Autodesk Inventor part; units mm, degrees
(part 2 of 2)
  line L486 (-92.9242, 137.6382) -> (-92.9242, 136.9026) construction
  line L487 (-92.9242, 136.9026) -> (-86.3376, 126.2158) construction
  line L488 (-86.3376, 126.2158) -> (-85.8147, 126.2158) construction
  line L489 (-85.8147, 126.2158) -> (-86.0963, 127.2615) construction
  line L490 (-86.0963, 127.2615) -> (-92.2499, 139.3275) construction
  line L491 (-92.2499, 139.3275) -> (-96.1914, 145.3604) construction
  line L492 (-96.1914, 145.3604) -> (-96.6339, 145.642) construction
  line L493 (-96.6339, 145.642) -> (-99.1677, 146.7681) construction
  line L494 (-99.1677, 146.7681) -> (-105.7825, 149.6506) construction
  spline S7 degree 4 poles (-105.7825, 149.6506) (-98.5638, 144.2366) (-96.1387, 141.0784) (-92.9242, 137.6382) (-92.9242, 136.9026) (-86.3376, 126.2158) (-85.8147, 126.2158) (-86.0963, 127.2615) (-92.2499, 139.3275) (-96.1914, 145.3604) (-96.6339, 145.642) (-99.1677, 146.7681) (-105.7825, 149.6506) knots 1 1 1 1 1 2 3 4 5 6 7 8 9 10 10 10 10 10
  line L495 (-151.4576, 116.9137) -> (-151.4576, 113.6219)
  line L496 (-232.8904, 100.9083) -> (-224.086, 105.444) construction
  line L497 (-224.086, 105.444) -> (-217.8517, 107.8081) construction
  line L498 (-217.8517, 107.8081) -> (-210.9325, 109.9735) construction
  line L499 (-210.9325, 109.9735) -> (-204.045, 111.8416) construction
  line L500 (-204.045, 111.8416) -> (-196.96, 113.1781) construction
  line L501 (-196.96, 113.1781) -> (-181.3524, 115.2983) construction
  line L502 (-181.3524, 115.2983) -> (-172.7322, 116.2018) construction
  line L503 (-172.7322, 116.2018) -> (-164.4787, 116.6804) construction
  line L504 (-164.4787, 116.6804) -> (-155.3689, 116.9137) construction
  line L505 (-155.3689, 116.9137) -> (-151.4576, 116.9137) construction
  spline S8 degree 4 poles (-232.8904, 100.9083) (-224.086, 105.444) (-217.8517, 107.8081) (-210.9325, 109.9735) (-204.045, 111.8416) (-196.96, 113.1781) (-181.3524, 115.2983) (-172.7322, 116.2018) (-164.4787, 116.6804) (-155.3689, 116.9137) (-151.4576, 116.9137) knots 1 1 1 1 1 2 3 4 5 6 7 8 8 8 8 8
  line L506 (-151.4576, 113.6219) -> (-160.6161, 113.6219) construction
  line L507 (-160.6161, 113.6219) -> (-167.753, 113.3145) construction
  line L508 (-167.753, 113.3145) -> (-176.028, 112.8336) construction
  line L509 (-176.028, 112.8336) -> (-190.3891, 111.4372) construction
  line L510 (-190.3891, 111.4372) -> (-200.0112, 109.6691) construction
  line L511 (-200.0112, 109.6691) -> (-210.3251, 107.9445) construction
  line L512 (-210.3251, 107.9445) -> (-217.922, 106.0369) construction
  line L513 (-217.922, 106.0369) -> (-223.8067, 104.1386) construction
  line L514 (-223.8067, 104.1386) -> (-227.183, 102.909) construction
  line L515 (-227.183, 102.909) -> (-229.6689, 101.9664) construction
  line L516 (-229.6689, 101.9664) -> (-232.2744, 101.1419) construction
  line L517 (-232.2744, 101.1419) -> (-232.8904, 100.9083) construction
  spline S9 degree 4 poles (-151.4576, 113.6219) (-160.6161, 113.6219) (-167.753, 113.3145) (-176.028, 112.8336) (-190.3891, 111.4372) (-200.0112, 109.6691) (-210.3251, 107.9445) (-217.922, 106.0369) (-223.8067, 104.1386) (-227.183, 102.909) (-229.6689, 101.9664) (-232.2744, 101.1419) (-232.8904, 100.9083) knots 1 1 1 1 1 2 3 4 5 6 7 8 9 10 10 10 10 10
  line L518 (-201.4615, 98.1456) -> (-198.4129, 100.8521) construction
  line L519 (-198.4129, 100.8521) -> (-196.3192, 102.3711) construction
  line L520 (-196.3192, 102.3711) -> (-194.2664, 103.5238) construction
  line L521 (-194.2664, 103.5238) -> (-191.3421, 104.8481) construction
  line L522 (-191.3421, 104.8481) -> (-187.3069, 106.5757) construction
  line L523 (-187.3069, 106.5757) -> (-184.015, 107.9604) construction
  line L524 (-184.015, 107.9604) -> (-181.0006, 109.0583) construction
  line L525 (-181.0006, 109.0583) -> (-179.1462, 109.7366) construction
  line L526 (-179.1462, 109.7366) -> (-174.5466, 111.2151) construction
  line L527 (-174.5466, 111.2151) -> (-172.2748, 111.8831) construction
  line L528 (-172.2748, 111.8831) -> (-171.1664, 112.1657) construction
  spline S10 degree 4 poles (-201.4615, 98.1456) (-198.4129, 100.8521) (-196.3192, 102.3711) (-194.2664, 103.5238) (-191.3421, 104.8481) (-187.3069, 106.5757) (-184.015, 107.9604) (-181.0006, 109.0583) (-179.1462, 109.7366) (-174.5466, 111.2151) (-172.2748, 111.8831) (-171.1664, 112.1657) knots 1 1 1 1 1 2 3 4 5 6 7 8 9 9 9 9 9
  line L529 (-171.1664, 112.1657) -> (-174.7868, 110.3396) construction
  line L530 (-174.7868, 110.3396) -> (-176.4505, 109.5236) construction
  line L531 (-176.4505, 109.5236) -> (-178.3607, 108.6636) construction
  line L532 (-178.3607, 108.6636) -> (-180.8153, 107.389) construction
  line L533 (-180.8153, 107.389) -> (-182.668, 106.5757) construction
  line L534 (-182.668, 106.5757) -> (-184.7906, 105.4752) construction
  line L535 (-184.7906, 105.4752) -> (-188.8328, 103.7438) construction
  line L536 (-188.8328, 103.7438) -> (-192.9088, 101.6116) construction
  line L537 (-192.9088, 101.6116) -> (-201.4615, 98.1456) construction
  spline S11 degree 4 poles (-171.1664, 112.1657) (-174.7868, 110.3396) (-176.4505, 109.5236) (-178.3607, 108.6636) (-180.8153, 107.389) (-182.668, 106.5757) (-184.7906, 105.4752) (-188.8328, 103.7438) (-192.9088, 101.6116) (-201.4615, 98.1456) knots 1 1 1 1 1 2 3 4 5 6 7 7 7 7 7
  line L538 (-175.3989, 90.8936) -> (-175.0678, 91.6636) construction
  line L539 (-167.9379, 100.2753) -> (-166.4649, 101.6772) construction
  line L540 (-166.4649, 101.6772) -> (-163.3138, 104.358) construction
  line L541 (-163.3138, 104.358) -> (-160.8042, 106.4947) construction
  line L542 (-160.8042, 106.4947) -> (-158.3215, 108.2959) construction
  line L543 (-158.3215, 108.2959) -> (-156.8552, 109.3592) construction
  line L544 (-156.8552, 109.3592) -> (-154.7761, 110.5531) construction
  spline S12 degree 4 poles (-175.3989, 90.8936) (-175.0678, 91.6636) (-174.5782, 92.4731) (-173.7131, 93.7871) (-171.7339, 96.3811) (-169.8583, 98.3242) (-167.9379, 100.2753) (-166.4649, 101.6772) (-163.3138, 104.358) (-160.8042, 106.4947) (-158.3215, 108.2959) (-156.8552, 109.3592) (-154.7761, 110.5531) knots 1 1 1 1 1 1.158039 1.166811 1.450335 2 3 4 5 6 7 7 7 7 7
  line L545 (-175.3989, 90.8936) -> (-172.1206, 94.0179) construction
  line L546 (-172.1206, 94.0179) -> (-168.4171, 97.5439) construction
  line L547 (-168.4171, 97.5439) -> (-165.0932, 101.0251) construction
  line L548 (-165.0932, 101.0251) -> (-161.4603, 104.2831) construction
  line L549 (-161.4603, 104.2831) -> (-159.6446, 105.8928) construction
  line L550 (-159.6446, 105.8928) -> (-157.3682, 108.0729) construction
  line L551 (-157.3682, 108.0729) -> (-154.7761, 110.5531) construction
  spline S13 degree 4 poles (-175.3989, 90.8936) (-172.1206, 94.0179) (-168.4171, 97.5439) (-165.0932, 101.0251) (-161.4603, 104.2831) (-159.6446, 105.8928) (-157.3682, 108.0729) (-154.7761, 110.5531) knots 1 1 1 1 1 2 3 4 5 5 5 5 5
  line L552 (-175.0678, 91.6636) -> (-174.5782, 92.4731) construction
  line L553 (-169.8583, 98.3242) -> (-167.9379, 100.2753) construction
  line L554 (-174.5782, 92.4731) -> (-173.7131, 93.7871) construction
  line L555 (-173.7131, 93.7871) -> (-171.7339, 96.3811) construction
  line L556 (-171.7339, 96.3811) -> (-169.8583, 98.3242) construction
  line L557 (-151.4576, 103.7438) -> (-159.2171, 103.7438) construction
  line L558 (-159.2171, 103.7438) -> (-161.5118, 103.8212) construction
  line L559 (-161.5118, 103.8212) -> (-165.7493, 103.995) construction
  line L560 (-165.7493, 103.995) -> (-174.3234, 104.7988) construction
  line L561 (-174.3234, 104.7988) -> (-183.963, 105.7115) construction
  line L562 (-183.963, 105.7115) -> (-192.1813, 106.8081) construction
  line L563 (-192.1813, 106.8081) -> (-200.9668, 108.2959) construction
  line L564 (-200.9668, 108.2959) -> (-205.9243, 109.313) construction
  spline S14 degree 4 poles (-151.4576, 103.7438) (-159.2171, 103.7438) (-161.5118, 103.8212) (-165.7493, 103.995) (-174.3234, 104.7988) (-183.963, 105.7115) (-192.1813, 106.8081) (-200.9668, 108.2959) (-205.9243, 109.313) knots 1 1 1 1 1 2 3 4 5 6 6 6 6 6
  line L565 (-205.9243, 109.313) -> (-206.0734, 108.8908) construction
  line L566 (-206.0734, 108.8908) -> (-205.7492, 108.8908) construction
  line L567 (-205.7492, 108.8908) -> (-204.6748, 108.4348) construction
  line L568 (-204.6748, 108.4348) -> (-201.8623, 107.6091) construction
  line L569 (-201.8623, 107.6091) -> (-199.298, 106.9147) construction
  line L570 (-199.298, 106.9147) -> (-194.7707, 106.0254) construction
  line L571 (-194.7707, 106.0254) -> (-191.951, 105.5403) construction
  line L572 (-191.951, 105.5403) -> (-189.8785, 105.1889) construction
  line L573 (-189.8785, 105.1889) -> (-183.7764, 104.1859) construction
  line L574 (-183.7764, 104.1859) -> (-176.1265, 103.3428) construction
  line L575 (-176.1265, 103.3428) -> (-169.656, 102.8387) construction
  line L576 (-169.656, 102.8387) -> (-165.7493, 102.5809) construction
  line L577 (-165.7493, 102.5809) -> (-160.6663, 102.3711) construction
  line L578 (-160.6663, 102.3711) -> (-154.8757, 102.2382) construction
  line L579 (-154.8757, 102.2382) -> (-151.4576, 102.2382) construction
  spline S15 degree 4 poles (-205.9243, 109.313) (-206.0734, 108.8908) (-205.7492, 108.8908) (-204.6748, 108.4348) (-201.8623, 107.6091) (-199.298, 106.9147) (-194.7707, 106.0254) (-191.951, 105.5403) (-189.8785, 105.1889) (-183.7764, 104.1859) (-176.1265, 103.3428) (-169.656, 102.8387) (-165.7493, 102.5809) (-160.6663, 102.3711) (-154.8757, 102.2382) (-151.4576, 102.2382) knots 1 1 1 1 1 2 3 4 5 6 7 8 9 10 11 12 13 13 13 13 13
  line L580 (-151.4576, 103.7438) -> (-151.4576, 102.2382)
  line L581 (-118.9522, 105.7115) -> (-110.734, 106.8081) construction
  spline S16 degree 4 poles (-151.4576, 103.7438) (-143.6982, 103.7438) (-141.4035, 103.8212) (-137.166, 103.995) (-128.5918, 104.7988) (-118.9522, 105.7115) (-110.734, 106.8081) (-101.9485, 108.2959) (-96.991, 109.313) knots 1 1 1 1 1 2 3 4 5 6 6 6 6 6
  line L582 (-151.4576, 103.7438) -> (-143.6982, 103.7438) construction
  line L583 (-143.6982, 103.7438) -> (-141.4035, 103.8212) construction
  line L584 (-141.4035, 103.8212) -> (-137.166, 103.995) construction
  line L585 (-137.166, 103.995) -> (-128.5918, 104.7988) construction
  line L586 (-128.5918, 104.7988) -> (-118.9522, 105.7115) construction
  line L587 (-110.734, 106.8081) -> (-101.9485, 108.2959) construction
  line L588 (-101.9485, 108.2959) -> (-96.991, 109.313) construction
  line L589 (-110.9642, 105.5403) -> (-113.0367, 105.1889) construction
  spline S17 degree 4 poles (-96.991, 109.313) (-96.8419, 108.8908) (-97.1661, 108.8908) (-98.2405, 108.4348) (-101.053, 107.6091) (-103.6172, 106.9147) (-108.1446, 106.0254) (-110.9642, 105.5403) (-113.0367, 105.1889) (-119.1389, 104.1859) (-126.7887, 103.3428) (-133.2593, 102.8387) (-137.166, 102.5809) (-142.249, 102.3711) (-148.0396, 102.2382) (-151.4576, 102.2382) knots 1 1 1 1 1 2 3 4 5 6 7 8 9 10 11 12 13 13 13 13 13
  line L590 (-96.991, 109.313) -> (-96.8419, 108.8908) construction
  line L591 (-96.8419, 108.8908) -> (-97.1661, 108.8908) construction
  line L592 (-97.1661, 108.8908) -> (-98.2405, 108.4348) construction
  line L593 (-98.2405, 108.4348) -> (-101.053, 107.6091) construction
  line L594 (-101.053, 107.6091) -> (-103.6172, 106.9147) construction
  line L595 (-103.6172, 106.9147) -> (-108.1446, 106.0254) construction
  line L596 (-108.1446, 106.0254) -> (-110.9642, 105.5403) construction
  line L597 (-113.0367, 105.1889) -> (-119.1389, 104.1859) construction
  line L598 (-119.1389, 104.1859) -> (-126.7887, 103.3428) construction
  line L599 (-126.7887, 103.3428) -> (-133.2593, 102.8387) construction
  line L600 (-133.2593, 102.8387) -> (-137.166, 102.5809) construction
  line L601 (-137.166, 102.5809) -> (-142.249, 102.3711) construction
  line L602 (-142.249, 102.3711) -> (-148.0396, 102.2382) construction
  line L603 (-148.0396, 102.2382) -> (-151.4576, 102.2382) construction
  spline S18 degree 4 poles (-151.4576, 113.6219) (-142.2991, 113.6219) (-135.1622, 113.3145) (-126.8873, 112.8336) (-112.5261, 111.4372) (-102.904, 109.6691) (-92.5902, 107.9445) (-84.9933, 106.0369) (-79.1085, 104.1386) (-75.7322, 102.909) (-73.2463, 101.9664) (-70.6409, 101.1419) (-70.0249, 100.9083) knots 1 1 1 1 1 2 3 4 5 6 7 8 9 10 10 10 10 10
  line L604 (-151.4576, 113.6219) -> (-142.2991, 113.6219) construction
  line L605 (-142.2991, 113.6219) -> (-135.1622, 113.3145) construction
  line L606 (-135.1622, 113.3145) -> (-126.8873, 112.8336) construction
  line L607 (-126.8873, 112.8336) -> (-112.5261, 111.4372) construction
  line L608 (-112.5261, 111.4372) -> (-102.904, 109.6691) construction
  line L609 (-102.904, 109.6691) -> (-92.5902, 107.9445) construction
  line L610 (-92.5902, 107.9445) -> (-84.9933, 106.0369) construction
  line L611 (-84.9933, 106.0369) -> (-79.1085, 104.1386) construction
  line L612 (-79.1085, 104.1386) -> (-75.7322, 102.909) construction
  line L613 (-75.7322, 102.909) -> (-73.2463, 101.9664) construction
  line L614 (-73.2463, 101.9664) -> (-70.6409, 101.1419) construction
  line L615 (-70.6409, 101.1419) -> (-70.0249, 100.9083) construction
  line L616 (-105.9552, 113.1781) -> (-121.5628, 115.2983) construction
  spline S19 degree 4 poles (-70.0249, 100.9083) (-78.8293, 105.444) (-85.0636, 107.8081) (-91.9828, 109.9735) (-98.8702, 111.8416) (-105.9552, 113.1781) (-121.5628, 115.2983) (-130.183, 116.2018) (-138.4365, 116.6804) (-147.5463, 116.9137) (-151.4576, 116.9137) knots 1 1 1 1 1 2 3 4 5 6 7 8 8 8 8 8
  line L617 (-70.0249, 100.9083) -> (-78.8293, 105.444) construction
  line L618 (-78.8293, 105.444) -> (-85.0636, 107.8081) construction
  line L619 (-85.0636, 107.8081) -> (-91.9828, 109.9735) construction
  line L620 (-91.9828, 109.9735) -> (-98.8702, 111.8416) construction
  line L621 (-98.8702, 111.8416) -> (-105.9552, 113.1781) construction
  line L622 (-121.5628, 115.2983) -> (-130.183, 116.2018) construction
  line L623 (-130.183, 116.2018) -> (-138.4365, 116.6804) construction
  line L624 (-138.4365, 116.6804) -> (-147.5463, 116.9137) construction
  line L625 (-147.5463, 116.9137) -> (-151.4576, 116.9137) construction
  spline S20 degree 4 poles (-131.7489, 112.1657) (-128.1284, 110.3396) (-126.4648, 109.5236) (-124.5546, 108.6636) (-122.1, 107.389) (-120.2473, 106.5757) (-118.1247, 105.4752) (-114.0825, 103.7438) (-110.0064, 101.6116) (-101.4537, 98.1456) knots 1 1 1 1 1 2 3 4 5 6 7 7 7 7 7
  line L626 (-131.7489, 112.1657) -> (-128.1284, 110.3396) construction
  line L627 (-128.1284, 110.3396) -> (-126.4648, 109.5236) construction
  line L628 (-126.4648, 109.5236) -> (-124.5546, 108.6636) construction
  line L629 (-124.5546, 108.6636) -> (-122.1, 107.389) construction
  line L630 (-122.1, 107.389) -> (-120.2473, 106.5757) construction
  line L631 (-120.2473, 106.5757) -> (-118.1247, 105.4752) construction
  line L632 (-118.1247, 105.4752) -> (-114.0825, 103.7438) construction
  line L633 (-114.0825, 103.7438) -> (-110.0064, 101.6116) construction
  line L634 (-110.0064, 101.6116) -> (-101.4537, 98.1456) construction
  line L635 (-118.9003, 107.9604) -> (-121.9147, 109.0583) construction
  spline S21 degree 4 poles (-101.4537, 98.1456) (-104.5024, 100.8521) (-106.596, 102.3711) (-108.6489, 103.5238) (-111.5731, 104.8481) (-115.6084, 106.5757) (-118.9003, 107.9604) (-121.9147, 109.0583) (-123.769, 109.7366) (-128.3687, 111.2151) (-130.6405, 111.8831) (-131.7489, 112.1657) knots 1 1 1 1 1 2 3 4 5 6 7 8 9 9 9 9 9
  line L636 (-101.4537, 98.1456) -> (-104.5024, 100.8521) construction
  line L637 (-104.5024, 100.8521) -> (-106.596, 102.3711) construction
  line L638 (-106.596, 102.3711) -> (-108.6489, 103.5238) construction
  line L639 (-108.6489, 103.5238) -> (-111.5731, 104.8481) construction
  line L640 (-111.5731, 104.8481) -> (-115.6084, 106.5757) construction
  line L641 (-115.6084, 106.5757) -> (-118.9003, 107.9604) construction
  line L642 (-121.9147, 109.0583) -> (-123.769, 109.7366) construction
  line L643 (-123.769, 109.7366) -> (-128.3687, 111.2151) construction
  line L644 (-128.3687, 111.2151) -> (-130.6405, 111.8831) construction
  line L645 (-130.6405, 111.8831) -> (-131.7489, 112.1657) construction
  spline S22 degree 4 poles (-127.5164, 90.8936) (-127.8475, 91.6636) (-128.337, 92.4731) (-129.2022, 93.7871) (-131.1813, 96.3811) (-133.057, 98.3242) (-134.9773, 100.2753) (-136.4504, 101.6772) (-139.6014, 104.358) (-142.1111, 106.4947) (-144.5937, 108.2959) (-146.0601, 109.3592) (-148.1391, 110.5531) knots 1 1 1 1 1 1.158039 1.166811 1.450335 2 3 4 5 6 7 7 7 7 7
  line L646 (-127.5164, 90.8936) -> (-127.8475, 91.6636) construction
  line L647 (-127.8475, 91.6636) -> (-128.337, 92.4731) construction
  line L648 (-128.337, 92.4731) -> (-129.2022, 93.7871) construction
  line L649 (-129.2022, 93.7871) -> (-131.1813, 96.3811) construction
  line L650 (-131.1813, 96.3811) -> (-133.057, 98.3242) construction
  line L651 (-133.057, 98.3242) -> (-134.9773, 100.2753) construction
  line L652 (-134.9773, 100.2753) -> (-136.4504, 101.6772) construction
  line L653 (-136.4504, 101.6772) -> (-139.6014, 104.358) construction
  line L654 (-139.6014, 104.358) -> (-142.1111, 106.4947) construction
  line L655 (-142.1111, 106.4947) -> (-144.5937, 108.2959) construction
  line L656 (-144.5937, 108.2959) -> (-146.0601, 109.3592) construction
  line L657 (-146.0601, 109.3592) -> (-148.1391, 110.5531) construction
  spline S23 degree 4 poles (-127.5164, 90.8936) (-130.7947, 94.0179) (-134.4982, 97.5439) (-137.822, 101.0251) (-141.4549, 104.2831) (-143.2707, 105.8928) (-145.5471, 108.0729) (-148.1391, 110.5531) knots 1 1 1 1 1 2 3 4 5 5 5 5 5
  line L658 (-127.5164, 90.8936) -> (-130.7947, 94.0179) construction
  line L659 (-130.7947, 94.0179) -> (-134.4982, 97.5439) construction
  line L660 (-134.4982, 97.5439) -> (-137.822, 101.0251) construction
  line L661 (-137.822, 101.0251) -> (-141.4549, 104.2831) construction
  line L662 (-141.4549, 104.2831) -> (-143.2707, 105.8928) construction
  line L663 (-143.2707, 105.8928) -> (-145.5471, 108.0729) construction
  line L664 (-145.5471, 108.0729) -> (-148.1391, 110.5531) construction
  line L665 (-224, 83) -> (-77, 83) construction
  line L666 (-77, 83) -> (-77, 71) construction
  line L667 (-77, 71) -> (-224, 71) construction
  line L668 (-224, 71) -> (-224, 83) construction
  line L669 (-314, -5) -> (18, -5) projected
  line L670 (-314, 353) -> (-314, -5) projected
  line L671 (18, -5) -> (18, 353) projected
  line L672 (-222.5563, 82.7921) -> (-211.9192, 82.7921)
  line L673 (-211.9192, 82.7921) -> (-211.9192, 80.2166)
  line L674 (-211.9192, 80.2166) -> (-218.2368, 80.2166)
  line L675 (-218.2368, 80.2166) -> (-218.2368, 78.1261)
  line L676 (-218.2368, 78.1261) -> (-212.8431, 78.1261)
  line L677 (-212.8431, 78.1261) -> (-212.8431, 75.7007)
  line L678 (-212.8431, 75.7007) -> (-218.2368, 75.7007)
  line L679 (-218.2368, 75.7007) -> (-218.2368, 70.7921)
  line L680 (-218.2368, 70.7921) -> (-222.5563, 70.7921)
  line L681 (-222.5563, 70.7921) -> (-222.5563, 82.7921)
  line L682 (-209.6092, 82.7921) -> (-205.3128, 82.7921)
  line L683 (-205.3128, 82.7921) -> (-205.3128, 73.7488)
  line L684 (-205.3128, 73.7488) -> (-198.591, 73.7488)
  line L685 (-198.591, 73.7488) -> (-198.591, 70.7921)
  line L686 (-198.591, 70.7921) -> (-209.6092, 70.7921)
  line L687 (-209.6092, 70.7921) -> (-209.6092, 82.7921)
  line L688 (-198.0481, 82.7921) -> (-193.2666, 82.7921)
  line L689 (-193.2666, 82.7921) -> (-190.4601, 78.7498)
  line L690 (-190.4601, 78.7498) -> (-187.642, 82.7921)
  line L691 (-187.642, 82.7921) -> (-182.8951, 82.7921)
  line L692 (-182.8951, 82.7921) -> (-188.3118, 75.8162)
  line L693 (-188.3118, 75.8162) -> (-188.3118, 70.7921)
  line L694 (-188.3118, 70.7921) -> (-192.6198, 70.7921)
  line L695 (-192.6198, 70.7921) -> (-192.6198, 75.8162)
  line L696 (-192.6198, 75.8162) -> (-198.0481, 82.7921)
  line L697 (-181.3359, 82.7921) -> (-177.0279, 82.7921)
  line L698 (-177.0279, 82.7921) -> (-177.0279, 70.7921)
  line L699 (-177.0279, 70.7921) -> (-181.3359, 70.7921)
  line L700 (-181.3359, 70.7921) -> (-181.3359, 82.7921)
  line L701 (-173.9095, 82.7921) -> (-169.8903, 82.7921)
  line L702 (-169.8903, 82.7921) -> (-164.6468, 76.1511)
  line L703 (-164.6468, 76.1511) -> (-164.6468, 82.7921)
  line L704 (-164.6468, 82.7921) -> (-160.5929, 82.7921)
  line L705 (-160.5929, 82.7921) -> (-160.5929, 70.7921)
  line L706 (-160.5929, 70.7921) -> (-164.6468, 70.7921)
  line L707 (-164.6468, 70.7921) -> (-169.8672, 77.3985)
  line L708 (-169.8672, 77.3985) -> (-169.8672, 70.7921)
  line L709 (-169.8672, 70.7921) -> (-173.9095, 70.7921)
  line L710 (-173.9095, 70.7921) -> (-173.9095, 82.7921)
  line L711 (-150.7411, 75.1347) -> (-150.7411, 77.6295)
  line L712 (-150.7411, 77.6295) -> (-144.0885, 77.6295)
  line L713 (-144.0885, 77.6295) -> (-144.0885, 72.5245)
  spline S24 degree 2 poles (-144.0885, 72.5245) (-145.9942, 71.3927) (-148.9278, 70.5842) (-150.949, 70.5842) knots 0 0 0 1 2 2 2
  spline S25 degree 2 poles (-150.949, 70.5842) (-153.4321, 70.5842) (-156.5505, 72.0395) (-158.2714, 74.9269) (-158.2714, 76.7979) knots 0 0 0 1 2 3 3 3
  spline S26 degree 2 poles (-158.2714, 76.7979) (-158.2714, 78.7613) (-156.3888, 81.6602) (-154.5756, 82.4225) knots 0 0 0 1 2 2 2
  spline S27 degree 2 poles (-154.5756, 82.4225) (-153.155, 83) (-150.7642, 83) knots 0 0 0 1 1 1
  spline S28 degree 2 poles (-150.7642, 83) (-148.4543, 83) (-146.1675, 82.2839) (-144.6545, 80.7594) (-144.2733, 79.6044) knots 0 0 0 1 2 3 3 3
  line L714 (-144.2733, 79.6044) -> (-148.4196, 78.9577)
  spline S29 degree 2 poles (-148.4196, 78.9577) (-148.6737, 79.6391) (-149.9095, 80.3667) (-150.8566, 80.3667) knots 0 0 0 1 2 2 2
  spline S30 degree 2 poles (-150.8566, 80.3667) (-152.2772, 80.3667) (-153.9634, 78.6689) (-153.9634, 76.8325) knots 0 0 0 1 2 2 2
  spline S31 degree 2 poles (-153.9634, 76.8325) (-153.9634, 74.8922) (-152.2541, 73.2175) (-150.7411, 73.2175) knots 0 0 0 1 2 2 2
  spline S32 degree 2 poles (-150.7411, 73.2175) (-150.0135, 73.2175) (-148.6968, 73.5756) (-147.8537, 74.0144) knots 0 0 0 1 2 2 2
  line L715 (-147.8537, 74.0144) -> (-147.8537, 75.1347)
  line L716 (-147.8537, 75.1347) -> (-150.7411, 75.1347)
  line L717 (-135.0337, 82.7921) -> (-126.9836, 82.7921)
  spline S33 degree 2 poles (-126.9836, 82.7921) (-124.974, 82.7921) (-122.8142, 81.0712) (-122.8142, 79.8008) knots 0 0 0 1 2 2 2
  spline S34 degree 2 poles (-122.8142, 79.8008) (-122.8142, 78.7382) (-123.5881, 77.9759) knots 0 0 0 1 1 1
  spline S35 degree 2 poles (-123.5881, 77.9759) (-124.0962, 77.4678) (-125.078, 77.1675) knots 0 0 0 1 1 1
  spline S36 degree 2 poles (-125.078, 77.1675) (-123.5881, 76.8556) (-122.1675, 75.3426) (-122.1675, 74.1992) knots 0 0 0 1 2 2 2
  spline S37 degree 2 poles (-122.1675, 74.1992) (-122.1675, 73.2753) (-123.1723, 71.7854) (-124.05, 71.3465) knots 0 0 0 1 2 2 2
  spline S38 degree 2 poles (-124.05, 71.3465) (-124.5929, 71.0808) (-125.6785, 70.9538) knots 0 0 0 1 1 1
  spline S39 degree 2 poles (-125.6785, 70.9538) (-127.1338, 70.7921) (-127.6073, 70.7921) knots 0 0 0 1 1 1
  line L718 (-127.6073, 70.7921) -> (-135.0337, 70.7921)
  line L719 (-135.0337, 70.7921) -> (-135.0337, 82.7921)
  line L720 (-130.691, 73.3677) -> (-128.4966, 73.3677)
  spline S40 degree 2 poles (-128.4966, 73.3677) (-127.3879, 73.3677) (-126.4755, 74.0491) (-126.4755, 74.615) knots 0 0 0 1 2 2 2
  spline S41 degree 2 poles (-126.4755, 74.615) (-126.4755, 75.1463) (-127.3763, 75.7931) (-128.5082, 75.7931) knots 0 0 0 1 2 2 2
  line L721 (-128.5082, 75.7931) -> (-130.691, 75.7931)
  line L722 (-130.691, 75.7931) -> (-130.691, 73.3677)
  line L723 (-130.691, 78.0799) -> (-128.82, 78.0799)
  spline S42 degree 2 poles (-128.82, 78.0799) (-127.8152, 78.0799) (-127.0298, 78.6805) (-127.0298, 79.2464) knots 0 0 0 1 2 2 2
  spline S43 degree 2 poles (-127.0298, 79.2464) (-127.0298, 79.7661) (-127.8152, 80.3551) (-128.7969, 80.3551) knots 0 0 0 1 2 2 2
  line L724 (-128.7969, 80.3551) -> (-130.691, 80.3551)
  line L725 (-130.691, 80.3551) -> (-130.691, 78.0799)
  line L726 (-119.9153, 82.7921) -> (-108.3888, 82.7921)
  line L727 (-108.3888, 82.7921) -> (-108.3888, 80.2281)
  line L728 (-108.3888, 80.2281) -> (-115.6073, 80.2281)
  line L729 (-115.6073, 80.2281) -> (-115.6073, 78.3224)
  line L730 (-115.6073, 78.3224) -> (-108.9086, 78.3224)
  line L731 (-108.9086, 78.3224) -> (-108.9086, 75.8739)
  line L732 (-108.9086, 75.8739) -> (-115.6073, 75.8739)
  line L733 (-115.6073, 75.8739) -> (-115.6073, 73.5063)
  line L734 (-115.6073, 73.5063) -> (-108.1809, 73.5063)
  line L735 (-108.1809, 73.5063) -> (-108.1809, 70.7921)
  line L736 (-108.1809, 70.7921) -> (-119.9153, 70.7921)
  line L737 (-119.9153, 70.7921) -> (-119.9153, 82.7921)
  line L738 (-97.3128, 72.7786) -> (-102.1983, 72.7786)
  line L739 (-102.1983, 72.7786) -> (-102.8797, 70.7921)
  line L740 (-102.8797, 70.7921) -> (-107.2801, 70.7921)
  line L741 (-107.2801, 70.7921) -> (-102.0481, 82.7921)
  line L742 (-102.0481, 82.7921) -> (-97.3359, 82.7921)
  line L743 (-97.3359, 82.7921) -> (-92.1155, 70.7921)
  line L744 (-92.1155, 70.7921) -> (-96.6198, 70.7921)
  line L745 (-96.6198, 70.7921) -> (-97.3128, 72.7786)
  line L746 (-98.2137, 75.3773) -> (-99.7382, 79.6853)
  line L747 (-99.7382, 79.6853) -> (-101.2627, 75.3773)
  line L748 (-101.2627, 75.3773) -> (-98.2137, 75.3773)
  line L749 (-90.6833, 70.7921) -> (-90.6833, 82.7921)
  line L750 (-90.6833, 82.7921) -> (-83.5111, 82.7921)
  spline S44 degree 2 poles (-83.5111, 82.7921) (-81.513, 82.7921) (-79.411, 82.2031) (-78.1174, 80.6092) (-78.1174, 79.4658) knots 0 0 0 1 2 3 3 3
  spline S45 degree 2 poles (-78.1174, 79.4658) (-78.1174, 78.461) (-79.1107, 77.0173) (-79.9653, 76.5669) knots 0 0 0 1 2 2 2
  spline S46 degree 2 poles (-79.9653, 76.5669) (-80.5197, 76.2782) (-81.4783, 76.0934) knots 0 0 0 1 1 1
  spline S47 degree 2 poles (-81.4783, 76.0934) (-80.7161, 75.8739) (-80.358, 75.6429) knots 0 0 0 1 1 1
  spline S48 degree 2 poles (-80.358, 75.6429) (-80.127, 75.5043) (-79.2262, 74.5342) (-79.076, 74.2685) knots 0 0 0 1 2 2 2
  line L751 (-79.076, 74.2685) -> (-76.9856, 70.7921)
  line L752 (-76.9856, 70.7921) -> (-81.8479, 70.7921)
  line L753 (-81.8479, 70.7921) -> (-84.1463, 74.4649)
  spline S49 degree 2 poles (-84.1463, 74.4649) (-84.5852, 75.1694) (-84.9317, 75.3888) knots 0 0 0 1 1 1
  spline S50 degree 2 poles (-84.9317, 75.3888) (-85.3936, 75.666) (-85.9827, 75.666) knots 0 0 0 1 1 1
  line L754 (-85.9827, 75.666) -> (-86.3638, 75.666)
  line L755 (-86.3638, 75.666) -> (-86.3638, 70.7921)
  line L756 (-86.3638, 70.7921) -> (-90.6833, 70.7921)
  line L757 (-86.3638, 77.9297) -> (-84.5505, 77.9297)
  spline S51 degree 2 poles (-84.5505, 77.9297) (-84.2502, 77.9297) (-83.4071, 78.0914) knots 0 0 0 1 1 1
  spline S52 degree 2 poles (-83.4071, 78.0914) (-82.9798, 78.1723) (-82.437, 78.7729) (-82.437, 79.1655) knots 0 0 0 1 2 2 2
  spline S53 degree 2 poles (-82.437, 79.1655) (-82.437, 79.743) (-83.2916, 80.3667) (-84.4697, 80.3667) knots 0 0 0 1 2 2 2
  line L758 (-84.4697, 80.3667) -> (-86.3638, 80.3667)
  line L759 (-86.3638, 80.3667) -> (-86.3638, 77.9297)
  point P0 (0, 0)
  point P1 (0, 0)
  dimension "d18" = 88
  dimension "d19" = 12
  dimension "d20" = 90
  dimension "d21" = 95
  constraints: 4 end point, 64 other
  measures "d18" distance between parallel lines of L669 L665
  measures "d19" distance between parallel lines of L667 L665
  measures "d20" distance between parallel lines of L670 L668
  measures "d21" distance between parallel lines of L671 L666
extrude "Выдавливание2" add sketch "Эскиз2" along normal blind 0.1 contours S0 | S19 S18 S17 S16 L495 | L495 S9 S14 S15 S8 | S14 S10 S15 S9 | S9 S15 S14 | S18 S17 S21 S16 | S16 S17 S18 | S14 S11 S15 S10 | S10 S11 S14 | S21 S17 S20 S16 | S16 S20 S21 | S15 S11 S10 | S21 S20 S17 | S14 S12 S15 S11 | S20 S17 S22 S16 | S14 S13 S15 S12 | S12 S13 S14 | S22 S17 S23 S16 | S16 S23 S22 | S15 S13 S12 | S22 S23 S17 | S14 L580 S15 S13 | S23 S17 L580 S16 | L672 L673 L674 L675 L676 L677 L678 L679 L680 L681 | L682 L683 L684 L685 L686 L687 | L688 L689 L690 L691 L692 L693 L694 L695 L696 | L697 L698 L699 L700 | L701 L702 L703 L704 L705 L706 L707 L708 L709 L710 | L711 L712 L713 S24 S25 S26 S27 S28 L714 S29 S30 S31 S32 L715 L716 | L717 S33 S34 S35 S36 S37 S38 S39 L718 L719 | L726 L727 L728 L729 L730 L731 L732 L733 L734 L735 L736 L737 | L738 L739 L740 L741 L742 L743 L744 L745 | L749 L750 S44 S45 S46 S47 S48 L751 L752 L753 S49 S50 L754 L755 L756
